Autodesk Inventor part; units mm, degrees
(part 3 of 3)
  spline S555 degree 2 poles (12.5558, 9.8472) (12.8066, 9.8472) (12.8066, 9.5964) knots 0 0 0 1 1 1
  line L569 (12.8066, 9.5964) -> (12.8066, 9.0156)
  spline S556 degree 2 poles (12.8066, 9.0156) (12.8066, 8.8769) (13.0013, 8.6822) (13.1366, 8.6822) knots 0 0 0 1 2 2 2
  line L570 (13.1366, 8.6822) -> (13.8594, 8.6822)
  spline S557 degree 2 poles (17.0772, 7.273) (17.0772, 7.0222) (16.8231, 7.0222) knots 0 0 0 1 1 1
  line L571 (16.8231, 7.0222) -> (15.8528, 7.0222)
  spline S558 degree 2 poles (15.8528, 7.0222) (15.5096, 7.0222) (15.0211, 7.5073) (15.0211, 7.8538) knots 0 0 0 1 2 2 2
  line L572 (15.0211, 7.8538) -> (15.0211, 9.5964)
  spline S559 degree 2 poles (15.0211, 9.5964) (15.0211, 9.8472) (15.2719, 9.8472) knots 0 0 0 1 1 1
  spline S560 degree 2 poles (15.2719, 9.8472) (15.5228, 9.8472) (15.5228, 9.5964) knots 0 0 0 1 1 1
  line L573 (15.5228, 9.5964) -> (15.5228, 7.8538)
  spline S561 degree 2 poles (15.5228, 7.8538) (15.5228, 7.7152) (15.7175, 7.5205) (15.8528, 7.5205) knots 0 0 0 1 2 2 2
  line L574 (15.8528, 7.5205) -> (16.5756, 7.5205)
  line L575 (16.5756, 7.5205) -> (16.5756, 9.5964)
  spline S562 degree 2 poles (16.5756, 9.5964) (16.5756, 9.8472) (16.8264, 9.8472) knots 0 0 0 1 1 1
  spline S563 degree 2 poles (16.8264, 9.8472) (17.0772, 9.8472) (17.0772, 9.5964) knots 0 0 0 1 1 1
  line L576 (17.0772, 9.5964) -> (17.0772, 7.273)
  line L577 (18.899, 9.3489) -> (18.2389, 9.3489)
  line L578 (18.2389, 9.3489) -> (18.2389, 7.273)
  spline S564 degree 2 poles (18.2389, 7.273) (18.2389, 7.0222) (17.9881, 7.0222) knots 0 0 0 1 1 1
  spline S565 degree 2 poles (17.9881, 7.0222) (17.7373, 7.0222) (17.7373, 7.273) knots 0 0 0 1 1 1
  line L579 (17.7373, 7.273) -> (17.7373, 9.5964)
  spline S566 degree 2 poles (17.7373, 9.5964) (17.7373, 9.8472) (17.9881, 9.8472) knots 0 0 0 1 1 1
  line L580 (17.9881, 9.8472) -> (19.7274, 9.8472)
  spline S567 degree 2 poles (19.7274, 9.8472) (20.0739, 9.8472) (20.5624, 9.3588) (20.5624, 9.0156) knots 0 0 0 1 2 2 2
  line L581 (20.5624, 9.0156) -> (20.5624, 7.273)
  spline S568 degree 2 poles (20.5624, 7.273) (20.5624, 7.0222) (20.3115, 7.0222) knots 0 0 0 1 1 1
  spline S569 degree 2 poles (20.3115, 7.0222) (20.0607, 7.0222) (20.0607, 7.273) knots 0 0 0 1 1 1
  line L582 (20.0607, 7.273) -> (20.0607, 9.0189)
  spline S570 degree 2 poles (20.0607, 9.0189) (20.0607, 9.1509) (19.8627, 9.3489) (19.7307, 9.3489) knots 0 0 0 1 2 2 2
  line L583 (19.7307, 9.3489) -> (19.4007, 9.3489)
  line L584 (19.4007, 9.3489) -> (19.4007, 7.273)
  spline S571 degree 2 poles (19.4007, 7.273) (19.4007, 7.0222) (19.1498, 7.0222) knots 0 0 0 1 1 1
  spline S572 degree 2 poles (19.1498, 7.0222) (18.899, 7.0222) (18.899, 7.273) knots 0 0 0 1 1 1
  line L585 (18.899, 7.273) -> (18.899, 9.3489)
  line L586 (21.7241, 8.6822) -> (22.4436, 8.6822)
  spline S573 degree 2 poles (22.4436, 8.6822) (22.8396, 8.6822) (23.0838, 8.372) knots 0 0 0 1 1 1
  spline S574 degree 2 poles (23.0838, 8.372) (23.2785, 8.1839) (23.2785, 7.8538) knots 0 0 0 1 1 1
  spline S575 degree 2 poles (23.2785, 7.8538) (23.2785, 7.5172) (23.0838, 7.372) knots 0 0 0 1 1 1
  spline S576 degree 2 poles (23.0838, 7.372) (22.8396, 7.0222) (22.4436, 7.0222) knots 0 0 0 1 1 1
  line L587 (22.4436, 7.0222) -> (21.4733, 7.0222)
  spline S577 degree 2 poles (21.4733, 7.0222) (21.2224, 7.0222) (21.2224, 7.273) knots 0 0 0 1 1 1
  line L588 (21.2224, 7.273) -> (21.2224, 9.5964)
  spline S578 degree 2 poles (21.2224, 9.5964) (21.2224, 9.8472) (21.4733, 9.8472) knots 0 0 0 1 1 1
  spline S579 degree 2 poles (21.4733, 9.8472) (21.7241, 9.8472) (21.7241, 9.5964) knots 0 0 0 1 1 1
  line L589 (21.7241, 9.5964) -> (21.7241, 8.6822)
  line L590 (21.7241, 8.1839) -> (21.7241, 7.5205)
  line L591 (21.7241, 7.5205) -> (22.4436, 7.5205)
  spline S580 degree 2 poles (22.4436, 7.5205) (22.602, 7.5205) (22.7571, 7.6393) knots 0 0 0 1 1 1
  spline S581 degree 2 poles (22.7571, 7.6393) (22.7769, 7.7152) (22.7769, 7.8538) knots 0 0 0 1 1 1
  spline S582 degree 2 poles (22.7769, 7.8538) (22.7769, 7.9892) (22.7604, 8.0651) knots 0 0 0 1 1 1
  spline S583 degree 2 poles (22.7604, 8.0651) (22.602, 8.1839) (22.4436, 8.1839) knots 0 0 0 1 1 1
  line L592 (22.4436, 8.1839) -> (21.7241, 8.1839)
  spline S584 degree 2 poles (-22.2755, -21.2988) (-22.3374, -21.3483) (-22.7335, -21.8228) knots 0 0 0 1 1 1
  line L593 (-22.7335, -21.8228) -> (-22.7335, -22.5695)
  spline S585 degree 2 poles (-22.7335, -22.5695) (-22.7335, -22.883) (-23.047, -22.883) knots 0 0 0 1 1 1
  spline S586 degree 2 poles (-23.047, -22.883) (-23.3605, -22.883) (-23.3605, -22.5695) knots 0 0 0 1 1 1
  line L594 (-23.3605, -22.5695) -> (-23.3605, -19.6652)
  spline S587 degree 2 poles (-23.3605, -19.6652) (-23.3605, -19.3516) (-23.047, -19.3516) knots 0 0 0 1 1 1
  spline S588 degree 2 poles (-23.047, -19.3516) (-22.7335, -19.3516) (-22.7335, -19.6652) knots 0 0 0 1 1 1
  line L595 (-22.7335, -19.6652) -> (-22.7335, -21.0224)
  line L596 (-22.7335, -21.0224) -> (-21.2731, -19.4135)
  spline S589 degree 2 poles (-21.2731, -19.4135) (-21.2359, -19.3393) (-21.1163, -19.3393) knots 0 0 0 1 1 1
  spline S590 degree 2 poles (-21.1163, -19.3393) (-20.9884, -19.3393) (-20.8028, -19.5455) (-20.8028, -19.6693) knots 0 0 0 1 2 2 2
  spline S591 degree 2 poles (-20.8028, -19.6693) (-20.8028, -19.8013) (-20.8976, -19.8962) knots 0 0 0 1 1 1
  line L597 (-20.8976, -19.8962) -> (-21.8506, -20.878)
  line L598 (-21.8506, -20.878) -> (-20.8729, -22.3673)
  spline S592 degree 2 poles (-20.8729, -22.3673) (-20.8028, -22.4746) (-20.8028, -22.5736) knots 0 0 0 1 1 1
  spline S593 degree 2 poles (-20.8028, -22.5736) (-20.8028, -22.7056) (-21.0008, -22.8912) (-21.1204, -22.8912) knots 0 0 0 1 2 2 2
  spline S594 degree 2 poles (-21.1204, -22.8912) (-21.2731, -22.8912) (-21.3184, -22.7964) knots 0 0 0 1 1 1
  line L599 (-21.3184, -22.7964) -> (-22.2755, -21.2988)
  spline S595 degree 2 poles (-17.3539, -22.5695) (-17.3539, -22.883) (-17.6675, -22.883) knots 0 0 0 1 1 1
  spline S596 degree 2 poles (-17.6675, -22.883) (-17.981, -22.883) (-17.981, -22.5695) knots 0 0 0 1 1 1
  line L600 (-17.981, -22.5695) -> (-17.981, -19.9746)
  line L601 (-17.981, -19.9746) -> (-18.4142, -19.9746)
  line L602 (-18.4142, -19.9746) -> (-19.3217, -22.718)
  spline S597 degree 2 poles (-19.3217, -22.718) (-19.3712, -22.883) (-19.5899, -22.883) knots 0 0 0 1 1 1
  spline S598 degree 2 poles (-19.5899, -22.883) (-19.9117, -22.883) (-19.9117, -22.5818) knots 0 0 0 1 1 1
  spline S599 degree 2 poles (-19.9117, -22.5818) (-19.9117, -22.5241) (-19.8952, -22.4704) knots 0 0 0 1 1 1
  line L603 (-19.8952, -22.4704) -> (-18.9175, -19.5167)
  spline S600 degree 2 poles (-18.9175, -19.5167) (-18.8679, -19.3516) (-18.641, -19.3516) knots 0 0 0 1 1 1
  line L604 (-18.641, -19.3516) -> (-17.6675, -19.3516)
  spline S601 degree 2 poles (-17.6675, -19.3516) (-17.3539, -19.3516) (-17.3539, -19.6652) knots 0 0 0 1 1 1
  line L605 (-17.3539, -19.6652) -> (-17.3539, -22.5695)
  line L606 (-15.8935, -20.8079) -> (-15.5552, -20.8079)
  line L607 (-15.5552, -20.8079) -> (-15.5552, -20.2468)
  spline S602 degree 2 poles (-15.5552, -20.2468) (-15.5552, -19.8797) (-15.0354, -19.3516) (-14.66, -19.3516) knots 0 0 0 1 2 2 2
  line L608 (-14.66, -19.3516) -> (-14.3712, -19.3516)
  spline S603 degree 2 poles (-14.3712, -19.3516) (-13.9958, -19.3516) (-13.4719, -19.8756) (-13.4719, -20.2468) knots 0 0 0 1 2 2 2
  line L609 (-13.4719, -20.2468) -> (-13.4719, -21.9878)
  spline S604 degree 2 poles (-13.4719, -21.9878) (-13.4719, -22.3632) (-13.9917, -22.883) (-14.3712, -22.883) knots 0 0 0 1 2 2 2
  line L610 (-14.3712, -22.883) -> (-14.66, -22.883)
  spline S605 degree 2 poles (-14.66, -22.883) (-15.0354, -22.883) (-15.5552, -22.3632) (-15.5552, -21.9919) knots 0 0 0 1 2 2 2
  line L611 (-15.5552, -21.9919) -> (-15.5552, -21.4308)
  line L612 (-15.5552, -21.4308) -> (-15.8935, -21.4308)
  line L613 (-15.8935, -21.4308) -> (-15.8935, -22.5695)
  spline S606 degree 2 poles (-15.8935, -22.5695) (-15.8935, -22.883) (-16.2071, -22.883) knots 0 0 0 1 1 1
  spline S607 degree 2 poles (-16.2071, -22.883) (-16.5206, -22.883) (-16.5206, -22.5695) knots 0 0 0 1 1 1
  line L614 (-16.5206, -22.5695) -> (-16.5206, -19.6652)
  spline S608 degree 2 poles (-16.5206, -19.6652) (-16.5206, -19.3516) (-16.2071, -19.3516) knots 0 0 0 1 1 1
  spline S609 degree 2 poles (-16.2071, -19.3516) (-15.8935, -19.3516) (-15.8935, -19.6652) knots 0 0 0 1 1 1
  line L615 (-15.8935, -19.6652) -> (-15.8935, -20.8079)
  line L616 (-14.099, -21.9919) -> (-14.099, -20.2427)
  spline S610 degree 2 poles (-14.099, -20.2427) (-14.099, -20.1355) (-14.2599, -19.9746) (-14.3712, -19.9746) knots 0 0 0 1 2 2 2
  line L617 (-14.3712, -19.9746) -> (-14.66, -19.9746)
  spline S611 degree 2 poles (-14.66, -19.9746) (-14.7714, -19.9746) (-14.9282, -20.1355) (-14.9282, -20.2427) knots 0 0 0 1 2 2 2
  line L618 (-14.9282, -20.2427) -> (-14.9282, -21.9919)
  spline S612 degree 2 poles (-14.9282, -21.9919) (-14.9282, -22.1033) (-14.7714, -22.26) (-14.66, -22.26) knots 0 0 0 1 2 2 2
  line L619 (-14.66, -22.26) -> (-14.3712, -22.26)
  spline S613 degree 2 poles (-14.3712, -22.26) (-14.2599, -22.26) (-14.099, -22.1033) (-14.099, -21.9919) knots 0 0 0 1 2 2 2
  line L620 (-10.7038, -20.8079) -> (-10.7038, -19.6652)
  spline S614 degree 2 poles (-10.7038, -19.6652) (-10.7038, -19.3516) (-10.3902, -19.3516) knots 0 0 0 1 1 1
  spline S615 degree 2 poles (-10.3902, -19.3516) (-10.0767, -19.3516) (-10.0767, -19.6652) knots 0 0 0 1 1 1
  line L621 (-10.0767, -19.6652) -> (-10.0767, -22.5695)
  spline S616 degree 2 poles (-10.0767, -22.5695) (-10.0767, -22.883) (-10.3902, -22.883) knots 0 0 0 1 1 1
  spline S617 degree 2 poles (-10.3902, -22.883) (-10.7038, -22.883) (-10.7038, -22.5695) knots 0 0 0 1 1 1
  line L622 (-10.7038, -22.5695) -> (-10.7038, -21.4308)
  line L623 (-10.7038, -21.4308) -> (-11.6031, -21.4308)
  spline S618 degree 2 poles (-11.6031, -21.4308) (-12.0321, -21.4308) (-12.6468, -20.8244) (-12.6468, -20.3912) knots 0 0 0 1 2 2 2
  line L624 (-12.6468, -20.3912) -> (-12.6468, -19.6652)
  spline S619 degree 2 poles (-12.6468, -19.6652) (-12.6468, -19.3516) (-12.3333, -19.3516) knots 0 0 0 1 1 1
  spline S620 degree 2 poles (-12.3333, -19.3516) (-12.0198, -19.3516) (-12.0198, -19.6652) knots 0 0 0 1 1 1
  line L625 (-12.0198, -19.6652) -> (-12.0198, -20.3912)
  spline S621 degree 2 poles (-12.0198, -20.3912) (-12.0198, -20.5645) (-11.7764, -20.8079) (-11.6072, -20.8079) knots 0 0 0 1 2 2 2
  line L626 (-11.6072, -20.8079) -> (-10.7038, -20.8079)
  point P0 (0, 0)
  point P1 (24.325, 67.4719)
  point P2 (0, 63.4719)
  point P3 (0, 75.4719)
  point P4 (10.5101, 51.0024)
  dimension "d17" = 7
  dimension "d19" = 7
  dimension "d20" = 14
  dimension "d21" = 1
  dimension "d22" = 1
  dimension "d25" = 20
  dimension "d32" = 20
  dimension "d37" = 17.5
  dimension "d38" = 12
  dimension "d39" = 6
  dimension "d85" = 40
  dimension "d86" = 2
  dimension "d88" = 19.5
  dimension "d89" = 12
  dimension "d90" = 16
  dimension "d91" = 6
  dimension "d92" = 6
  dimension "d93" = 13
  dimension "d94" = 13
  dimension "d95" = 25
  dimension "d96" = 2
  dimension "d99" = 1
  dimension "d100" = 1
  dimension "d101" = 1
  dimension "d102" = 6
  dimension "d103" = 17
  dimension "d104" = 13
  dimension "d105" = 19.5
  dimension "d106" = 12
  dimension "d107" = 10
  dimension "d108" = 2
  dimension "d109" = 2
  dimension "d111" = 1
  dimension "d112" = 45
  dimension "d113" = 24
  dimension "d114" = 61
  dimension "d115" = 37
  dimension "d116" = 194
  dimension "d117" = 2
  dimension "d118" = 1
  constraints: 170 end point, 115 point on circle, 66 centre point, 44 tangent, 32 parallel, 21 perpendicular, 14 equal radius, 13 horizontal, 6 coincident, 5 vertical, 2 midpoint, 2 point on line, 1 symmetric about line, 133 other
  measures "d17" diameter of A0
  measures "d19" distance from line of L5 A0.centre
  measures "d20" distance between parallel lines of L4 L6
  measures "d21" radius of A1
  measures "d22" distance between parallel lines of L6 L7
  measures "d25" distance of A0.centre A9.centre
  measures "d32" distance of L7.end L31.end
  measures "d37" distance between parallel lines of L43 L41
  measures "d38" distance between parallel lines of L42 L40
  measures "d39" distance between parallel lines of L8 L40
  measures "d85" distance between parallel lines of L43 L49
  measures "d86" radius of A27
  measures "d88" distance between parallel lines of L61 L63
  measures "d89" distance between parallel lines of L62 L60
  measures "d90" distance from line of L55 point (10.51, 51.002)
  measures "d91" diameter of A35
  measures "d92" diameter of A36
  measures "d93" diameter of A37
  measures "d94" diameter of A38
  measures "d95" distance of A36.centre A35.centre
  measures "d96" radius of A39
  measures "d99" distance between parallel lines of L54 L51
  measures "d100" distance between parallel lines of L52 L53
  measures "d101" distance between parallel lines of L74 L81
  measures "d102" diameter of A47
  measures "d103" diameter of A48
  measures "d104" distance from line of L85 A47.centre
  measures "d105" distance between parallel lines of L100 L102
  measures "d106" distance between parallel lines of L101 L99
  measures "d107" distance between parallel lines of L92 L99
  measures "d108" radius of A49
  measures "d109" radius of A50
  measures "d111" distance between parallel lines of L84 L87
  measures "d112" distance between parallel lines of L114 L116
  measures "d113" distance between parallel lines of L115 L113
  measures "d114" distance between parallel lines of L117 L115
  measures "d115" diameter of A57
  measures "d116" distance from line of L128 A57.centre
  measures "d117" radius of A58
  measures "d118" distance between parallel lines of L129 L133
extrude "Выдавливание2" cut sketch "Эскиз2" against normal blind 10 contours A0 L44 | L44 A0 | A9 | A23 | L40 L41 L42 L43
extrude "Выдавливание3" add sketch "Эскиз2" along normal blind 2 contours L5 A3 L4 A2 L15 A7 L9 A6 L8 L44 | L44 L8 A5 L7 A8 L10 A1 L6 A4 L5 | L243 S166 L244 S167 L245 L44 L246 L247 L239 L240 L241 L242 | L44 L242 S164 S165 L243 | S117 S118 S119 S120 S121 S122 S123 S124 S125 L209 S126 S127 S128 S129 L44 S113 S114 S115 L208 | L44 L208 S116 S117 | L44 S129 S110 S111 S112 S113 | L195 L196 S98 S99 L197 S90 S91 L190 L191 S92 S93 L192 L44 | L44 L192 L193 S94 S95 L194 S96 S97 L195 | L44 L239 S162 S163 L240 | L44 L245 S168 S169 L246 | A10 L20 A11 L19 A13 L18 A16 L23 A15 L21 A14 L22 A17 L17 A12 L16 | L31 A20 L33 A21 L30 A19 L32 A22 L34 A24 L35 A25 L28 A26 L29 A18 | L137 S0 S1 L138 S2 S3 L139 L140 L141 S4 S5 L142 S6 S7 L143 L144 | L145 S8 L146 S9 L147 S10 S11 L148 S12 L149 S13 L150 S14 S15 | S16 S17 L151 L152 S18 S19 S20 L153 S21 S22 L154 | L155 L156 S23 S24 L157 S25 S26 L158 S27 S28 S29 S30 S31 S32 S33 S34 S35 | S36 L159 S37 L160 S38 S39 L161 S40 L162 S41 L163 S42 S43 L164 | S44 S45 S46 S47 S48 S49 L165 S50 S51 S52 S53 S54 S55 S56 S57 S58 S59 L166 S60 S61 S62 S63 | S64 L167 S65 L168 S66 L169 S67 S68 S69 | L176 S74 L177 S75 L178 S76 S77 L179 S78 L180 S79 L181 S80 S81 | S82 L182 S83 L183 S84 L184 S85 L185 | S100 L198 S101 L199 S102 L200 S103 S104 L201 S105 L202 S106 L203 L204 L205 S107 S108 L206 S109 L207 | S130 S131 L210 L211 S132 S133 L212 L213 S134 S135 L214 S136 S137 L215 L216 S138 S139 L217 | L218 S140 S141 S142 L219 S143 S144 L220 S145 S146 S147 L221 L222 | L226 S148 S149 L227 S150 S151 L228 L229 L230 S152 S153 L231 S154 S155 L232 L233 | L234 S156 S157 L235 S158 S159 L236 L237 S160 S161 L238 | L248 S170 S171 L249 S172 S173 L250 L251 L252 S174 S175 L253 S176 S177 L254 L255 | L256 S178 S179 L257 S180 S181 L258 L259 L260 S182 S183 L261 S184 S185 L262 L263 | S186 L264 S187 L265 S188 S189 L266 L267 S190 L268 | S193 S194 L273 S195 S196 L274
extrude "Выдавливание4" add sketch "Эскиз2" along normal blind 2 contours L275 S197 L276 S198 S199 L277 L278 S200 S201 | S202 L279 S203 L280 S204 L281 S205 L282 | S210 L287 S211 S212 S213 L288 L289 L290 S214 S215 L291 S216 L292 S217 | L296 S220 S221 S222 L297 S223 S224 L298 S225 S226 S227 L299 L300
sketch "Эскиз3" plane through (0, 0, 2) normal (0, 0, 1) x (1, 0, 0)
  point P0 (0, 0)
extrude "Выдавливание5" cut sketch "Эскиз2" against normal blind 2 contours L40 L41 L42 L43
extrude "Выдавливание7" [suppressed]
extrude "Выдавливание9" add sketch "Эскиз2" along normal blind 2 contours L74 A28 L50 A29 L51 L44 L54 A33 L55 A34 L81 | L44 L81 L80 L74 | L51 A30 L52 A27 L73 L72 L75 A31 L53 A32 L54 L44 | L304 S228 L305 S229 L306 S230 S231 L307 S232 L308 S233 L309 S234 S235 | S236 L310 S237 L311 S238 L312 S239 S240 S241 | S246 S247 L319 L320 L321 S248 S249 S250 L322 S251 L323 S252 L324 S253 L325 | S256 L330 S257 S258 S259 S260 S261 L331 S262 L332 S263 L333 S264 S265 L334 S266 S267 S268 S269 S270 S271 S272 S273 S274 S275 L335 | S276 L336 S277 L337 S278 S279 L338 L339 S280 L340
extrude "Выдавливание10" add sketch "Эскиз2" along normal blind 2 contours L447 L448 S404 S405 L449 S398 S399 L444 L44 | L44 L444 L445 S400 S401 L446 S402 S403 L447 | L345 S283 L346 S284 S285 L347 L348 S286 S287 | S288 L349 S289 L350 S290 L351 S291 L352 | S296 L357 S297 S298 S299 L358 L359 L360 S300 S301 L361 S302 L362 S303 | L366 S306 S307 S308 L367 S309 S310 L368 S311 S312 S313 L369 L370 | L374 S314 S315 L375 L376 S316 S317 L377 S318 S319 S320 L378 L379 S321 S322 L380 L381 S323 S324 S325 | S326 S327 L382 S328 S329 L383 | S330 L384 S331 S332 S333 L385 L386 L387 S334 S335 L388 S336 L389 S337 | L393 S340 S341 L394 L395 L396 S342 S343 L397 S344 L398 S345 L399 S346 S347 L400 L401 | L402 S348 S349 L403 L404 S350 S351 L405 S352 S353 S354 L406 L407 S355 S356 L408 L409 S357 S358 S359 | S360 S361 L410 S362 S363 L411 | S364 L412 S365 S366 S367 L413 L414 L415 S368 S369 L416 S370 L417 S371 | L421 S374 S375 L422 L423 L424 S376 S377 L425 S378 L426 S379 L427 S380 S381 L428 L429 | L430 S382 L431 S383 L432 S384 S385 L433 S386 L434 S387 L435 S388 S389 | S390 L436 S391 L437 S392 L438 S393 L439 | S406 S407 L450 L451 S408 S409 L452 S410 S411 L453 L454 S412 S413 L455 | L456 S414 S415 L457 L458 L459 S416 S417 L460 S418 L461 S419 L462 S420 S421 L463 L464 | L465 S422 L466 S423 L467 S424 S425 L468 S426 L469 S427 L470 S428 S429 | L471 S430 S431 L472 S432 S433 L473 L474 S434 S435 L475 | S436 S437 L476 S438 S439 L477 | S440 L478 S441 L479 S442 L480 S443 L481 | S448 S449 L486 L487 S450 S451 L488 S452 S453 L489 L490 S454 S455 L491 | S456 S457 L492 S458 L493 L494 S459 S460 L495 S461 L496 S462 L497 | L498 S463 L499 S464 S465 L500 S466 L501 L502 S467 S468 L503 S469 L504 S470 S471 L505 S472 L506 | S473 S474 L507 L508 L509 S475 S476 S477 L510 S478 L511 S479 L512 | L513 S480 S481 S482 S483 L514 S484 L515 S485 S486 L516 | L520 L521 S491 S492 L522 S493 L523 S494 L524 S495 S496 L525 S497 L526 L527 S498 S499 L528 | S500 S501 L529 S502 L530 S503 L531 S504 S505 S506 S507 S508 | S519 L537 S520 S521 L538 S522 S523 L539 L540 S524 S525 S526 L541 L542 S527 S528 S529 L543 | S530 S531 L544 L545 L546 S532 S533 S534 L547 S535 L548 S536 L549 | L550 L551 S537 L552 S538 L553 S539 L554 S540 L555 L556 L557 S541 S542 L558 S543 S544 L559 | L564 S549 S550 L565 S551 S552 L566 L567 S553 L568 S554 S555 L569 S556 L570 | S557 L571 S558 L572 S559 S560 L573 S561 L574 L575 S562 S563 L576 | L577 L578 S564 S565 L579 S566 L580 S567 L581 S568 S569 L582 S570 L583 L584 S571 S572 L585 | L586 S573 S574 S575 S576 L587 S577 L588 S578 S579 L589 | S584 L593 S585 S586 L594 S587 S588 L595 L596 S589 S590 S591 L597 L598 S592 S593 S594 L599 | S595 S596 L600 L601 L602 S597 S598 S599 L603 S600 L604 S601 L605 | L606 L607 S602 L608 S603 L609 S604 L610 S605 L611 L612 L613 S606 S607 L614 S608 S609 L615 | L620 S614 S615 L621 S616 S617 L622 L623 S618 L624 S619 S620 L625 S621 L626
extrude "Выдавливание11" cut sketch "Эскиз2" against normal blind 2 contours L60 L61 L62 L44 | L44 L62 L63 L60 | L113 L114 L115 L44 | L44 L115 L116 L113 | A57 L44 | L44 A57 | A35 | A36 | A47 | L99 L100 L101 L102
extrude "Выдавливание12" add sketch "Эскиз2" along normal blind 2 contours L123 A52 L107 A51 L108 L44 L111 A55 L112 A56 L120 | L44 L120 L119 L123 | L91 A42 L83 A41 L84 L44 L87 A45 L88 A46 L92 | L44 L92 L98 L91 | L44 L84 A40 L85 A39 L90 L89 L93 A43 L86 A44 L87 | L44 L108 A50 L109 A49 L122 L118 L121 A53 L110 A54 L111
